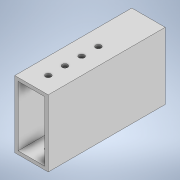
# Autodesk Inventor part: Part14
Saved by Autodesk Inventor 2022 (Build 260153000, 153)
## iProperties
Created: 2022-12-05
Part Number: Part14
Material: Generic
Document SubType Name: Modeling
Designer: s135320
Density: 1 g/cm^3
Appearance: Default
Author: s135320
Autodesk Inventor part; units mm, degrees
ref_plane "YZ Plane" through (0, 0, 0) normal (1, 0, 0) x (0, 1, 0)
ref_plane "XZ Plane" through (0, 0, 0) normal (0, 1, 0) x (-1, 0, 0)
ref_plane "XY Plane" through (0, 0, 0) normal (0, 0, 1) x (1, 0, 0)
sketch "Sketch1" plane through (0, 0, 0) normal (0, 1, 0) x (-1, 0, 0)
  line L0 (0, 0) -> (25.4, 0)
  line L1 (25.4, 0) -> (25.4, -88.9)
  line L2 (25.4, -88.9) -> (0, -88.9)
  line L3 (0, -88.9) -> (0, 0)
  dimension "d0" = 88.9
  dimension "d1" = 25.4
  constraints: 8 end point, 2 parallel, 1 horizontal, 1 perpendicular
  measures "d0" distance of L0.end L1.end
  measures "d1" distance of L1.end L2.end
extrude "Extrusion1" add sketch "Sketch1" along normal blind 50.8
shell "Shell1" thickness 2.54 removed faces 2 at (-16.9333, 33.8667, 0) at (-8.4667, 16.9333, -88.9)
sketch "Sketch2" plane through (0, 50.8, 0) normal (0, 1, 0) x (1, 0, 0)
  line L0 (-2.54, 0) -> (-22.86, 0) construction
  line L1 (-12.7, 0) -> (-12.7, 62.6675) construction
  circle A0 centre (-12.7, 0) radius 2.0701
  circle A1 centre (-12.7, 12.7) radius 2.0701
  circle A2 centre (-12.7, 25.4) radius 2.0701
  circle A3 centre (-12.7, 38.1) radius 2.0701
  circle A4 centre (-12.7, 50.8) radius 2.0701
  point P0 (0, 0)
  dimension "d5" = 4.1402
  dimension "d8" = 12.7
  constraints: 5 centre point, 2 end point, 1 coincident, 1 midpoint, 1 perpendicular, 1 vertical, 8 other
  measures "d5" diameter of A0
  measures "d8" distance of A0.centre A1.centre
extrude "Extrusion2" cut sketch "Sketch2" against normal through all contours A1 | A2 | A3 | A4
body "Solid1"
